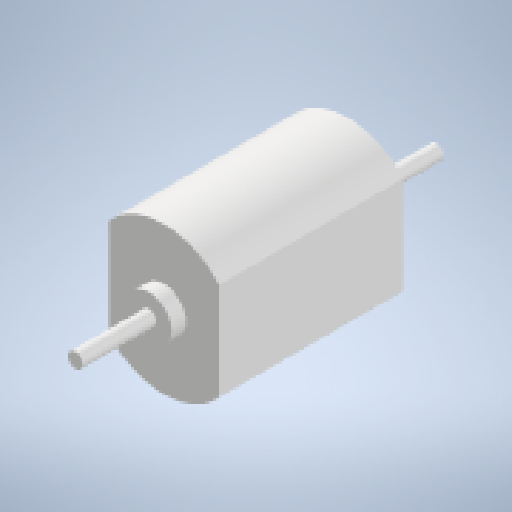
# Autodesk Inventor part: Motor_400
Saved by Autodesk Inventor 2024.1 (Build 281209000, 209)
## iProperties
Created: 2024-07-01
Part Number: Motor_400
Material: 一般
Document SubType Name: Modeling
Designer: hibik
Density: 1 g/cm^3
Appearance: 既定
Author: hibik
Autodesk Inventor part; units mm, degrees
ref_plane "YZ Plane" through (0, 0, 0) normal (1, 0, 0) x (0, 1, 0)
ref_plane "XZ Plane" through (0, 0, 0) normal (0, 1, 0) x (-1, 0, 0)
sketch "スケッチ1" plane through (0, 0, 0) normal (0, 0, 1) x (1, 0, 0)
  circle A0 centre (0, 0) radius 10
  line L0 (-7.5, 6.6144) -> (7.5, 6.6144) construction
  line L1 (7.5, 6.6144) -> (7.5, -6.6144)
  line L2 (7.5, -6.6144) -> (-7.5, -6.6144) construction
  line L3 (-7.5, -6.6144) -> (-7.5, 6.6144)
  dimension "d0" = 20
  dimension "d1" = 15
  constraints: 8 end point, 3 point on circle, 2 parallel, 1 centre point, 1 coincident, 1 horizontal, 1 perpendicular
  measures "d0" diameter of A0
  measures "d1" distance of L0.start L0.end
extrude "押し出し1" add sketch "スケッチ1" along normal blind 25 contours L1 A0 L3
sketch "スケッチ2" plane through (0, 0, 25) normal (0, 0, 1) x (1, 0, 0)
  circle A0 centre (0, 0) radius 3
  dimension "d4" = 6
  constraints: 1 centre point, 1 coincident
  measures "d4" diameter of A0
extrude "押し出し2" add sketch "スケッチ2" along normal blind 2
sketch "スケッチ3" plane through (0, 0, 0) normal (0, 0, -1) x (-1, 0, 0)
  circle A0 centre (0, 0) radius 5
  dimension "d7" = 10
  constraints: 1 centre point, 1 coincident
  measures "d7" diameter of A0
extrude "押し出し3" add sketch "スケッチ3" along normal blind 2
ref_plane "作業平面1" through (0, 0, -12) normal (0, 0, -1) x (-1, 0, 0)
sketch "スケッチ4" plane through (0, 0, -12) normal (0, 0, -1) x (-1, 0, 0)
  circle A0 centre (0, 0) radius 1
  dimension "d11" = 2
  constraints: 1 centre point, 1 coincident
  measures "d11" diameter of A0
extrude "押し出し4" add sketch "スケッチ4" against normal blind 49
